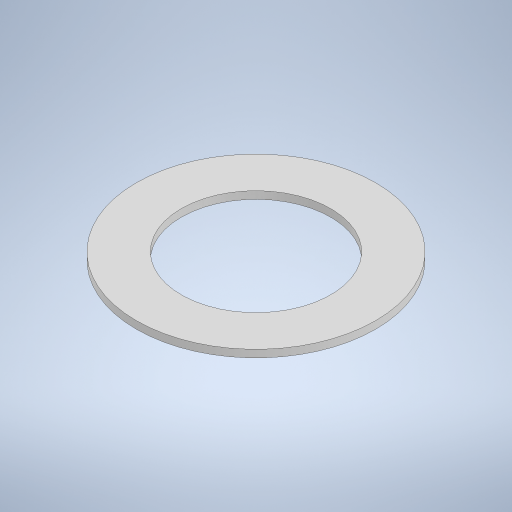
# Autodesk Inventor part: Shim
Saved by Autodesk Inventor 2023 (Build 270158030, 158C)
## iProperties
Created: 2022-10-01
Part Number: Shim
Material: Generic
Document SubType Name: Modeling
Designer: cjj5381
Density: 1 g/cm^3
Appearance: Default
Author: cjj5381
Autodesk Inventor part; units mm, degrees
ref_plane "YZ Plane" through (0, 0, 0) normal (1, 0, 0) x (0, 1, 0)
ref_plane "XZ Plane" through (0, 0, 0) normal (0, 1, 0) x (-1, 0, 0)
ref_plane "XY Plane" through (0, 0, 0) normal (0, 0, 1) x (1, 0, 0)
sketch "Sketch2" plane through (0, 0, 0) normal (0, 1, 0) x (-1, 0, 0)
  circle A0 centre (0, 0) radius 5
  circle A1 centre (0, 0) radius 8
  dimension "d0" = 10
  dimension "d1" = 16
  constraints: 2 centre point, 2 coincident
  measures "d0" diameter of A0
  measures "d1" diameter of A1
extrude "Extrusion1" add sketch "Sketch2" along normal blind 0.5
body "Solid1"
